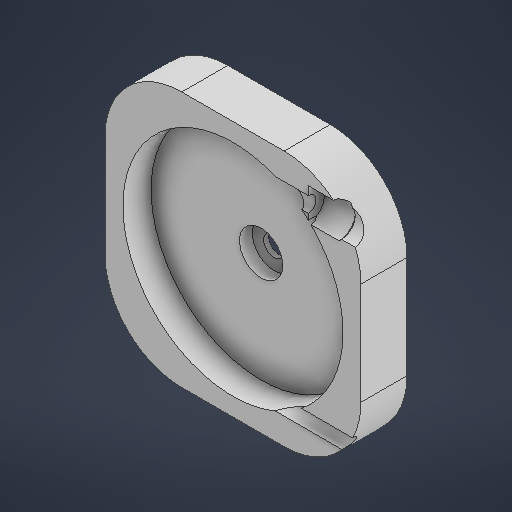
# Autodesk Inventor part: Case
Saved by Autodesk Inventor 2025.3 (Build 293356030, 356C)
## iProperties
Created: 2025-10-02
Part Number: Case
Material: Generic
Document SubType Name: Modeling
Designer: yo
Density: 1 g/cm^3
Appearance: Default
Author: yo
Autodesk Inventor part; units mm, degrees
ref_plane "YZ Plane" through (0, 0, 0) normal (1, 0, 0) x (0, 1, 0)
ref_plane "XZ Plane" through (0, 0, 0) normal (0, 1, 0) x (-1, 0, 0)
ref_plane "XY Plane" through (0, 0, 0) normal (0, 0, 1) x (1, 0, 0)
sketch "Sketch1" plane through (0, 0, 0) normal (0, 0, 1) x (1, 0, 0)
  line L0 (-20, 50) -> (20, 50)
  line L1 (50, 20) -> (50, -20)
  line L2 (20, -50) -> (-20, -50)
  line L3 (-50, -20) -> (-50, 20)
  circle A0 centre (0, 0) radius 43
  circle A1 centre (0, 0) radius 8.45
  circle A2 centre (0, 0) radius 4
  arc A3 (50, 20) -> (20, 50) centre (20, 20) ccw
  arc A4 (20, -50) -> (50, -20) centre (20, -20) ccw
  arc A5 (-50, -20) -> (-20, -50) centre (-20, -20) ccw
  arc A6 (-20, 50) -> (-50, 20) centre (-20, 20) ccw
  point P0 (-50, 50)
  point P1 (50, -50)
  point P2 (50, 50)
  point P3 (-50, -50)
  point P4 (0, 50)
  point P5 (50, 0)
  dimension "d0" = 100
  dimension "d1" = 86
  dimension "d2" = 16.9
  dimension "d3" = 8
  dimension "d10" = 30
  constraints: 8 end point, 8 point on circle, 8 point on line, 8 tangent, 7 centre point, 3 coincident, 3 equal radius, 2 midpoint, 2 parallel, 2 perpendicular, 1 horizontal, 1 horizontal alignment, 1 vertical alignment
  measures "d0" distance of point (-50, 50) point (50, 50)
  measures "d1" diameter of A0
  measures "d2" diameter of A1
  measures "d3" diameter of A2
  measures "d10" radius of A3
extrude "Extrusion1" add sketch "Sketch1" along normal blind 2 contours A1
extrude "Extrusion2" add sketch "Sketch1" along normal blind 7 contours A0
extrude "Extrusion3" add sketch "Sketch1" along normal blind 18 contours L0 A3 L1 A4 L2 A5 L3 A6
sketch "Sketch3" plane through (0, 0, 18) normal (0, 0, 1) x (1, 0, 0)
  circle A0 centre (0, 0) radius 43 projected
  line L0 (22.4487, 36.675) -> (65.4487, 36.675)
  line L1 (42.4487, 42) -> (48.4487, 42)
  line L2 (50.4487, 44) -> (65.4487, 44)
  line L3 (41.4487, 43) -> (29.4487, 43)
  line L4 (50.4487, 44) -> (48.4487, 42)
  line L5 (41.4487, 43) -> (42.4487, 42)
  line L6 (48.4487, 42) -> (65.4487, 42) construction
  line L7 (42.4487, 42) -> (29.4487, 42) construction
  line L8 (65.4487, 44) -> (65.4487, 36.675)
  line L9 (29.4487, 39.675) -> (22.4487, 39.675)
  line L10 (29.4487, 39.675) -> (29.4487, 43)
  line L11 (22.4487, 39.675) -> (22.4487, 36.675) construction
  line L12 (22.4487, 36.675) -> (16.5799, 36.675)
  line L13 (22.4487, 39.675) -> (16.5799, 39.675)
  line L14 (16.5799, 36.675) -> (16.5799, 39.675)
  circle A1 centre (0, 0) radius 4 projected
  line L15 (0, 0) -> (50, 0)
  line L16 (50, -20) -> (50, 20) projected
  line L17 (22.4487, -36.675) -> (65.4487, -36.675)
  line L18 (42.4487, -42) -> (48.4487, -42)
  line L19 (50.4487, -44) -> (65.4487, -44)
  line L20 (41.4487, -43) -> (29.4487, -43)
  line L21 (50.4487, -44) -> (48.4487, -42)
  line L22 (41.4487, -43) -> (42.4487, -42)
  line L23 (48.4487, -42) -> (65.4487, -42) construction
  line L24 (42.4487, -42) -> (29.4487, -42) construction
  line L25 (65.4487, -44) -> (65.4487, -36.675)
  line L26 (29.4487, -39.675) -> (22.4487, -39.675)
  line L27 (29.4487, -39.675) -> (29.4487, -43)
  line L28 (22.4487, -39.675) -> (22.4487, -36.675) construction
  line L29 (22.4487, -36.675) -> (16.5799, -36.675)
  line L30 (22.4487, -39.675) -> (16.5799, -39.675)
  line L31 (16.5799, -36.675) -> (16.5799, -39.675)
  line L32 (29.4487, -39.675) -> (65.4487, -39.675)
  dimension "d12" = 10.65
  dimension "d13" = 14.65
  dimension "d14" = 12.65
  dimension "d15" = 45
  dimension "d16" = 45
  dimension "d17" = 15
  dimension "d18" = 6
  dimension "d19" = 12
  dimension "d21" = 7
  dimension "d22" = 6
  constraints: 64 end point, 14 symmetric about line, 9 horizontal, 4 vertical, 4 vertical alignment, 2 point on circle, 1 midpoint, 1 perpendicular, 1 point on line, 1 tangent
  measures "d12" diameter of L1 L0
  measures "d13" diameter of L2 L0
  measures "d14" diameter of L3 L0
  measures "d15" angle of L6 L4
  measures "d16" angle of L5 L7
  measures "d17" distance of L2.start L2.end
  measures "d18" distance of L1.start L1.end
  measures "d19" distance of L3.start L3.end
  measures "d21" distance of L9.start L9.end
  measures "d22" diameter of L9 L0
revolve "Revolution1" cut sketch "Sketch3" angle 360 about axis through (22.4487, 36.675, 18) along (1, 0, 0) contours A0 L13 L9 L10 L3 L5 L1 L4 L2 L8 L0
revolve "Revolution2" cut sketch "Sketch3" angle 360 about axis through (22.4487, -36.675, 18) along (1, 0, 0) contours L17 L25 L32 L26 L30 A0
body "Solid1"
